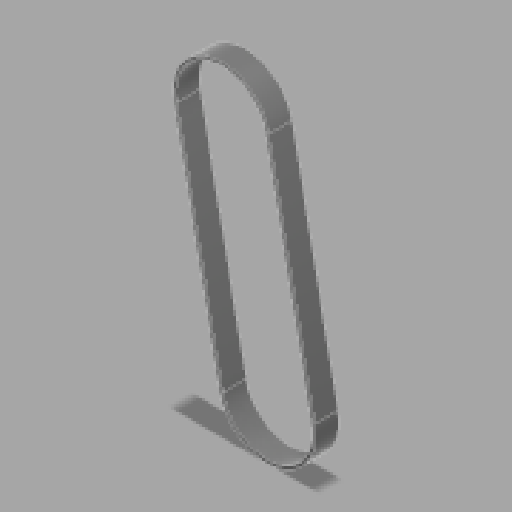
# Autodesk Inventor part: Ремень
Saved by Autodesk Inventor 2025 (Build 290162000, 162)
## iProperties
Created: 2025-04-08
Part Number: Ремень
Material: Типовые
Document SubType Name: Modeling
Designer: Artem Sannikov
Density: 1 g/cm^3
Appearance: Гладкая — черная
Author: Artem Sannikov
Autodesk Inventor part; units mm, degrees
ref_plane "YZ Plane" through (0, 0, 0) normal (1, 0, 0) x (0, 1, 0)
ref_plane "XZ Plane" through (0, 0, 0) normal (0, 1, 0) x (-1, 0, 0)
ref_plane "XY Plane" through (0, 0, 0) normal (0, 0, 1) x (1, 0, 0)
sketch "Эскиз1" plane through (0, 0, 0) normal (0, 0, 1) x (1, 0, 0)
  spline S0 degree 3 number of poles 571 construction
  circle A0 centre (0, 0) radius 12.4728
  circle A1 centre (0, 0) radius 11.6873
  spline S1 degree 3 number of poles 571 construction
  circle A2 centre (-11.8104, 58.8262) radius 3.05 construction
  circle A3 centre (-11.8104, 58.8262) radius 12.4622
  circle A4 centre (-11.8104, 58.8262) radius 11.6915
  line L0 (0.2776, 61.9276) -> (12.2284, 2.4573)
  line L1 (-24.0292, 56.3753) -> (-12.2292, -2.453)
  line L2 (-23.273, 56.524) -> (-11.4585, -2.3013)
  line L3 (-10.6007, -6.5724) -> (-10.5969, -6.5911)
  line L4 (-0.3475, 61.1267) -> (11.4588, 2.2997)
  point P0 (0.4075, 61.2814)
  dimension "d0" = 24.9244
  dimension "d1" = 24.9457
  dimension "d2" = 23.383
  dimension "d3" = 23.3746
  constraints: 10 end point, 8 tangent, 7 point on circle, 4 coincident, 3 centre point, 7 other
  measures "d1" diameter of A0
  measures "d2" diameter of A4
  measures "d3" diameter of A1
extrude "Выдавливание1" add sketch "Эскиз1" along normal blind 6 contours A0 L2 A1 L4 | A0 L4 A3 L0 | A3 L4 A4 L2 | L1 A3 L2 A0 picked at (-11.2889, -3.7346) picked at (-14.656, 70.613)
